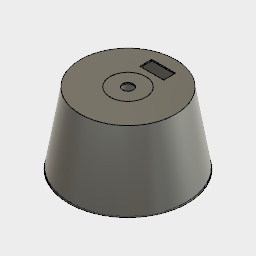
Top shell v4 (Autodesk Fusion 360 design; units mm, degrees)
Autodesk Fusion 360 part; units mm, degrees
sketch "Sketch1" plane through (0, 0, 0) normal (0, 1, 0) x (1, 0, 0)
  circle A0 centre (0, 0) radius 25
  dimension "d1" = 50
  measures "d1" diameter of A0
ref_plane "WorkPlane1" through (0, 30, 0) normal (0, 1, 0) x (1, 0, 0)
sketch "Sketch2" plane through (0, 30, 0) normal (0, 1, 0) x (1, 0, 0)
  circle A0 centre (0, 0) radius 20
  dimension "d3" = 40
  measures "d3" diameter of A0
loft "Loft1" add profiles "Sketch2", "Sketch1" section 1 section 2 makes body 1
shell "Shell1" thickness 0.5 removed faces 0 bodies 1
sketch "Sketch3" plane through (0, 0, 0) normal (0, 1, 0) x (1, 0, 0)
  circle A0 centre (0, 0) radius 24.75
  dimension "d5" = 49.5
  measures "d5" diameter of A0
extrude "Extrude1" cut sketch "Sketch3" along normal blind 0.5 bodies 1
cylinder "CylinderPrimitive1" add diameter 15 height -19 placed x (1, 0, 0) y (0, 0, -1) z (0, 1, 0) at (0, 30, 0) bodies 1
delete_face "DeleteFace1" 2 faces at (7.4627, 23.3333, 0.7468) (1.9158, 11, -2.8099) on bodies 1
sketch "Sketch5" plane through (0, 30, 0) normal (0, 1, 0) x (-1, 0, 0)
  circle A0 centre (0, 0) radius 20
  circle A1 centre (0, 0) radius 7.5
  dimension "d10" = 15
  measures "d10" diameter of A1
extrude "Extrude2" add sketch "Sketch5" against normal blind 19 contours A1 bodies 1
cylinder "CylinderPrimitive2" add diameter 15 height -19 placed x (1, 0, 0) y (0, 0, -1) z (0, 1, 0) at (0, 30, 0) separate body makes body 2
shell "Shell2" thickness 0.5 removed faces 0 bodies 2
sketch "Sketch7" plane through (0, 30, 0) normal (0, 1, 0) x (-1, 0, 0)
  circle A0 centre (0, 0) radius 7.5
  circle A1 centre (0, 0) radius 2.25
  dimension "d16" = 4.5
  measures "d16" diameter of A1
extrude "Extrude3" cut sketch "Sketch7" against normal blind 30 contours A1 bodies 1 2
sketch "Sketch8" plane through (0, 30, 0) normal (0, 1, 0) x (-1, 0, 0)
  circle A0 centre (0, 0) radius 2.25
  circle A1 centre (0, 0) radius 20
  line L0 (5, -15) -> (-5, -15)
  line L1 (-5, -15) -> (-5, -10)
  line L2 (-5, -10) -> (5, -10)
  line L3 (5, -10) -> (5, -15)
extrude "Extrude4" cut sketch "Sketch8" against normal blind 2 contours L0 L1 L2 L3 bodies 1
